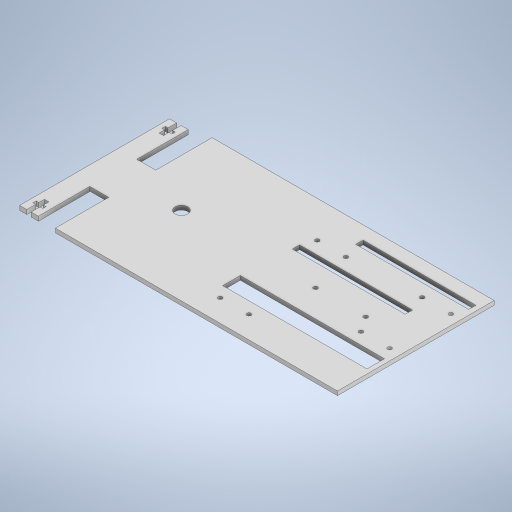
# Autodesk Inventor part: suelo_imp
Saved by Autodesk Inventor 2024 (Build 280153020, 153B)
## iProperties
Created: 2023-05-01
Part Number: suelo_imp
Material: Generic
Document SubType Name: Modeling
Designer: Diego
Density: 1 g/cm^3
Appearance: Default
Author: Diego
Autodesk Inventor part; units mm, degrees
ref_plane "YZ Plane" through (0, 0, 0) normal (1, 0, 0) x (0, 1, 0)
ref_plane "XZ Plane" through (0, 0, 0) normal (0, 1, 0) x (-1, 0, 0)
ref_plane "XY Plane" through (0, 0, 0) normal (0, 0, 1) x (1, 0, 0)
sketch "Sketch1" plane through (0, 0, 0) normal (0, 1, 0) x (-1, 0, 0)
  line L0 (-97.5, -62.5) -> (97.5, -62.5)
  line L1 (97.5, 62.5) -> (-97.5, 62.5)
  line L2 (-97.5, 62.5) -> (-97.5, -62.5)
  line L3 (-97.5, -62.5) -> (97.5, 62.5) construction
  line L4 (97.5, -62.5) -> (-97.5, 62.5) construction
  line L5 (97.5, 20) -> (112.525, 20)
  line L6 (127.475, 21.2237) -> (127.475, -18.7763)
  line L7 (112.525, -17.5526) -> (97.5, -17.5526)
  line L8 (97.5, -62.5) -> (97.5, -17.5526)
  line L9 (97.5, 20) -> (97.5, 62.5)
  line L10 (112.525, 20) -> (112.525, 61)
  line L11 (127.475, 61) -> (127.475, 21.2237)
  line L12 (127.475, 1.2237) -> (97.475, 1.2237) construction
  line L13 (112.525, -17.5526) -> (112.525, -58.5526)
  line L14 (127.475, -58.5526) -> (127.475, -18.7763)
  line L15 (119.975, 61) -> (121.775, 61) construction
  line L16 (118.225, 61) -> (118.225, 59)
  line L17 (119.975, 61) -> (119.975, 52.3078) construction
  line L18 (118.225, 59) -> (114.175, 59)
  line L19 (114.175, 59) -> (114.175, 56)
  line L20 (114.175, 56) -> (118.175, 56)
  line L21 (118.175, 56) -> (118.175, 53)
  line L22 (112.525, 61) -> (118.225, 61)
  line L23 (127.475, 61) -> (121.775, 61)
  line L24 (119.975, -58.5526) -> (121.775, -58.5526) construction
  line L25 (112.525, -58.5526) -> (118.225, -58.5526)
  line L26 (127.475, -58.5526) -> (121.775, -58.5526)
  line L27 (118.175, 53) -> (118.175, 47)
  line L28 (118.175, 47) -> (121.775, 47)
  line L29 (119.975, -58.5526) -> (121.775, -58.5526) construction
  line L30 (121.775, -58.5526) -> (121.775, -56.5526)
  line L31 (118.225, -58.5526) -> (118.225, -56.5526)
  line L32 (121.775, -56.5526) -> (125.775, -56.5526)
  line L33 (125.775, -56.5526) -> (125.775, -53.5526)
  line L34 (125.775, -53.5526) -> (121.775, -53.5526)
  line L35 (121.775, -58.5526) -> (121.775, -50.5526) construction
  line L36 (119.975, -58.5526) -> (119.975, -49.8604) construction
  line L37 (114.175, -53.5526) -> (118.175, -53.5526)
  line L38 (114.175, -56.5526) -> (114.175, -53.5526)
  line L39 (118.225, -56.5526) -> (114.175, -56.5526)
  line L40 (118.175, -53.5526) -> (118.175, -50.5526)
  line L41 (112.525, -58.5526) -> (118.225, -58.5526)
  line L42 (127.475, -58.5526) -> (121.775, -58.5526)
  line L43 (121.775, -53.5526) -> (121.775, -44.5526)
  line L44 (118.175, -50.5526) -> (118.175, -44.5526)
  line L45 (118.175, -44.5526) -> (121.775, -44.5526)
  line L46 (127.475, 61) -> (127.475, 79) construction
  line L47 (-97.5, 0) -> (-67.5, 0) construction
  line L48 (-67.5, 62.5) -> (-67.5, -62.5) construction
  line L49 (127.475, 79) -> (-67.5, 0) construction
  line L50 (127.475, -58.5526) -> (127.475, -76.5526) construction
  line L51 (127.475, -76.5526) -> (-67.5, 0) construction
  line L52 (-97.5, 62.5) -> (-117.5, 62.5)
  line L53 (-117.5, 62.5) -> (-117.5, -62.5)
  line L54 (-117.5, -62.5) -> (-97.5, -62.5)
  line L55 (-97.5, -62.5) -> (-97.5, 62.5)
  line L56 (-67.5, 0) -> (-47.5, 0) construction
  circle A0 centre (-47.5, 0) radius 1.6
  line L57 (-67.5, 0) -> (-87.5, 0) construction
  circle A1 centre (-87.5, 0) radius 1.6
  line L58 (121.775, 59.5898) -> (118.225, 59.5898) construction
  line L59 (121.775, 61) -> (121.775, 47)
  line L60 (121.775, 61) -> (121.775, 55) construction
  point P0 (0, 0)
  point P1 (121.775, 53)
  point P2 (121.775, -50.5526)
  point P3 (-97.5, -62.5)
  dimension "d0" = 195
  dimension "d1" = 125
  dimension "d3" = 30
  dimension "d4" = 40
  dimension "d5" = 15
  dimension "d6" = 41
  dimension "d11" = 7.5
  dimension "d12" = 1.8
  dimension "d13" = 1.75
  dimension "d15" = 2
  dimension "d21" = 30
  dimension "d22" = 8.6922
  dimension "d23" = 1.5
  dimension "d28" = 18
  dimension "d29" = 30
  dimension "d30" = 18
  dimension "d35" = 20
  dimension "d36" = 125
  dimension "d41" = 20
  dimension "d42" = 3.2
  dimension "d43" = 20
  dimension "d47" = 3.2
  dimension "d90" = 6
  constraints: 122 end point, 16 symmetric about line, 12 perpendicular, 7 horizontal, 7 point on line, 5 parallel, 5 vertical, 4 midpoint, 2 centre point, 2 coincident
  measures "d0" distance of L1.end L1.start
  measures "d1" distance of L1.start L0.end
  measures "d3" distance of L5.start L6.start
  measures "d4" distance of L6.start L6.end
  measures "d5" distance of L5.end L6.start
  measures "d6" distance of L5.end L10.end
  measures "d11" distance of L11.start L15.start
  measures "d12" distance of L15.end L15.start
  measures "d13" distance of L15.start L16.start
  measures "d15" distance of L16.start L16.end
  measures "d21" distance from line of L12.end L11
  measures "d22" distance from line of L17.end L23
  measures "d23" distance between parallel lines of L23 L1
  measures "d28" distance of L11.start L46.end
  measures "d29" distance of L47.start L47.end
  measures "d30" distance of L14.start L50.end
  measures "d35" distance of L54.end L53.end
  measures "d36" distance of L53.end L52.end
  measures "d41" distance of L47.end L56.end
  measures "d42" diameter of A0
  measures "d43" distance of L47.end L57.end
  measures "d47" diameter of A1
  measures "d90" distance of L15.end L60.end
extrude "Extrusion1" add sketch "Sketch1" along normal blind 3.25 contours L2 L1 L9 L5 L10 L22 L16 L18 L19 L20 L21 L27 L28 L59 L23 L11 L6 L14 L26 L30 L32 L33 L34 L43 L45 L44 L40 L37 L38 L39 L31 L25 L13 L7 L8 L0 | A0 | A1
sketch "Sketch2" plane through (0, 3.25, 0) normal (0, 1, 0) x (1, 0, 0)
  line L0 (-127.475, 58.5526) -> (-127.475, -61) construction
  line L1 (-127.475, 0) -> (-59.475, 0) construction
  circle A0 centre (-59.475, 0) radius 5
  point P0 (0, 0)
  dimension "d31" = 68
  dimension "d32" = 10
  constraints: 2 end point, 1 centre point, 1 coincident, 1 perpendicular, 1 point on line
  measures "d31" distance of L1.start L1.end
  measures "d32" diameter of A0
extrude "Extrusion2" cut sketch "Sketch2" against normal blind 10
sketch "Sketch3" plane through (97.5, 0, 62.5) normal (1, 0, 0) x (0, 0, -1)
  line L0 (125, 0) -> (80.0526, 0) projected
  line L1 (0, 3.25) -> (125, 3.25)
  line L2 (125, 3.25) -> (125, 0)
  line L3 (125, 0) -> (0, 0)
  line L4 (0, 0) -> (0, 3.25)
  point P0 (62.5, 0)
  constraints: 8 end point, 2 parallel, 1 horizontal, 1 perpendicular
extrude "Extrusion4" add sketch "Sketch3" along normal blind 30
extrude "Extrusion5" cut sketch "Sketch1" along normal blind 4 contours A0 | A1
sketch "Sketch4" plane through (0, 3.25, 0) normal (0, 1, 0) x (1, 0, 0)
  line L0 (-97.5, -62.5) -> (127.5, -62.5) construction
  line L1 (39.3, -62.5) -> (39.3, -44.9) construction
  line L2 (127.5, 62.5) -> (127.5, -62.5) construction
  circle A0 centre (39.3, -44.9) radius 1.6
  circle A1 centre (16.42, -44.9) radius 1.6
  line L3 (39.3, -44.9) -> (16.42, -44.9) construction
  line L4 (118.8, -62.5) -> (118.8, -12.2) construction
  circle A2 centre (118.8, -12.2) radius 1.6
  line L5 (118.8, -12.2) -> (95.92, -12.2) construction
  circle A3 centre (95.92, -12.2) radius 1.6
  line L6 (-97.5, 62.5) -> (127.5, 62.5) construction
  line L7 (119.5, 62.5) -> (119.5, 35.9) construction
  circle A4 centre (119.5, 35.9) radius 1.6
  line L8 (119.5, 35.9) -> (96.62, 35.9) construction
  circle A5 centre (96.62, 35.9) radius 1.6
  line L9 (38.32, 62.5) -> (38.32, 33.4) construction
  circle A6 centre (38.32, 33.4) radius 1.6
  line L10 (38.32, 33.4) -> (15.44, 33.4) construction
  circle A7 centre (15.44, 33.4) radius 1.6
  point P0 (0, 0)
  point P1 (119.5, 49.2)
  dimension "d48" = 88.2
  dimension "d49" = 17.6
  dimension "d50" = 3.2
  dimension "d51" = 3.2
  dimension "d52" = 22.88
  dimension "d53" = 50.3
  dimension "d54" = 8.7
  dimension "d55" = 3.2
  dimension "d56" = 3.2
  dimension "d57" = 22.88
  dimension "d58" = 8
  dimension "d59" = 26.6
  dimension "d60" = 3.2
  dimension "d61" = 22.88
  dimension "d62" = 3.2
  dimension "d63" = 89.18
  dimension "d64" = 29.1
  dimension "d65" = 3.2
  dimension "d66" = 22.88
  dimension "d67" = 3.2
  constraints: 16 end point, 8 centre point, 7 coincident, 4 point on line, 3 horizontal, 3 vertical, 2 perpendicular, 1 midpoint
  measures "d48" distance between parallel lines of L1 L2
  measures "d49" distance of L1.start L1.end
  measures "d50" diameter of A0
  measures "d51" diameter of A1
  measures "d52" distance of L3.start L3.end
  measures "d53" distance of L4.start L4.end
  measures "d54" distance between parallel lines of L2 L4
  measures "d55" diameter of A2
  measures "d56" diameter of A3
  measures "d57" distance of L5.start L5.end
  measures "d58" distance from line of L2 point (119.5, 49.2)
  measures "d59" distance of L7.start L7.end
  measures "d60" diameter of A4
  measures "d61" distance of L8.start L8.end
  measures "d62" diameter of A5
  measures "d63" distance between parallel lines of L2 L9
  measures "d64" distance of L9.start L9.end
  measures "d65" diameter of A6
  measures "d66" distance of L10.start L10.end
  measures "d67" diameter of A7
extrude "Extrusion6" cut sketch "Sketch4" against normal blind 10
sketch "Sketch5" plane through (0, 3.25, 0) normal (0, 1, 0) x (1, 0, 0)
  circle A0 centre (119.5, 35.9) radius 1.6 construction
  line L0 (123.5, 48.9829) -> (78.5, 48.9829) construction
  line L1 (123.5, 46.1029) -> (33.5, 46.1029)
  line L2 (33.5, 46.1029) -> (33.5, 51.8629)
  line L3 (33.5, 51.8629) -> (123.5, 51.8629)
  line L4 (123.5, 51.8629) -> (123.5, 46.1029)
  line L5 (123.5, 46.1029) -> (33.5, 51.8629) construction
  line L6 (33.5, 46.1029) -> (123.5, 51.8629) construction
  line L7 (127.5, 62.5) -> (127.5, -62.5) projected
  circle A1 centre (15.44, 33.4) radius 1.6 construction
  line L8 (11.5, 20.4) -> (56.5, 20.4) construction
  line L9 (101.5, 17.525) -> (11.5, 17.525)
  line L10 (11.5, 17.525) -> (11.5, 23.275)
  line L11 (11.5, 23.275) -> (101.5, 23.275)
  line L12 (101.5, 23.275) -> (101.5, 17.525)
  line L13 (101.5, 17.525) -> (11.5, 23.275) construction
  line L14 (11.5, 17.525) -> (101.5, 23.275) construction
  circle A2 centre (95.92, -12.2) radius 1.6 construction
  line L15 (111.5, -28.5) -> (66.5, -28.5) construction
  line L16 (124, -35.5) -> (9, -35.5)
  line L17 (9, -35.5) -> (9, -21.5)
  line L18 (9, -21.5) -> (124, -21.5)
  line L19 (124, -21.5) -> (124, -35.5)
  line L20 (124, -35.5) -> (9, -21.5) construction
  line L21 (9, -35.5) -> (124, -21.5) construction
  line L22 (-97.5, -62.5) -> (127.5, -62.5) projected
  point P0 (0, 0)
  dimension "d71" = 45
  dimension "d72" = 90
  dimension "d73" = 5.76
  dimension "d76" = 4
  dimension "d78" = 45
  dimension "d79" = 90
  dimension "d80" = 5.75
  dimension "d82" = 26
  dimension "d84" = 45
  dimension "d85" = 115
  dimension "d86" = 14
  dimension "d87" = 3.5
  dimension "d88" = 27
  constraints: 42 end point, 6 horizontal, 6 midpoint, 6 parallel, 3 perpendicular
  measures "d71" distance of L0.start L0.end
  measures "d72" distance of L2.end L3.end
  measures "d73" distance of L1.end L2.end
  measures "d76" distance between parallel lines of L7 L4
  measures "d78" distance of L8.start L8.end
  measures "d79" distance of L10.end L11.end
  measures "d80" distance of L9.end L10.end
  measures "d82" distance between parallel lines of L7 L12
  measures "d84" distance of L15.start L15.end
  measures "d85" distance of L17.end L18.end
  measures "d86" distance of L16.end L17.end
  measures "d87" distance between parallel lines of L7 L19
  measures "d88" distance between parallel lines of L16 L22
extrude "Extrusion7" cut sketch "Sketch5" against normal blind 10
sketch "Sketch6" plane through (0, 3.25, 0) normal (0, 1, 0) x (1, 0, 0)
  line L0 (-127.475, -61) -> (-121.775, -61) projected
  line L1 (-112.525, 17.5526) -> (-112.525, 58.5526) projected
  line L2 (-127.475, -61) -> (-112.525, -61)
  line L3 (-112.525, -61) -> (-112.525, 58.5526)
  line L4 (-112.525, 58.5526) -> (-127.475, 58.5526)
  line L5 (-127.475, 58.5526) -> (-127.475, -61)
  point P0 (0, 0)
  constraints: 8 end point, 2 parallel, 1 horizontal, 1 perpendicular
extrude "Extrusion8" add sketch "Sketch6" against normal blind 3.5
sketch "Sketch7" plane through (0, 3.25, 0) normal (0, 1, 0) x (1, 0, 0)
  line L0 (-112.525, -61) -> (-127.475, -61) construction
  line L1 (-120, -61) -> (-121.75, -61) construction
  line L2 (-120, -61) -> (-118.25, -61) construction
  line L3 (-121.75, -47) -> (-118.25, -47)
  line L4 (-120, -61) -> (-120, -55.8389) construction
  line L5 (-121.75, -54) -> (-123.95, -54)
  line L6 (-123.95, -54) -> (-123.95, -51.4)
  line L7 (-123.95, -51.4) -> (-121.75, -51.4)
  line L8 (-121.75, -61) -> (-121.75, -54)
  line L9 (-121.75, -51.4) -> (-121.75, -47)
  line L10 (-118.25, -47) -> (-121.75, -47)
  line L11 (-118.25, -54) -> (-116.05, -54)
  line L12 (-116.05, -54) -> (-116.05, -51.4)
  line L13 (-116.05, -51.4) -> (-118.25, -51.4)
  line L14 (-118.25, -61) -> (-118.25, -54)
  line L15 (-118.25, -51.4) -> (-118.25, -47)
  line L16 (-127.475, 58.5526) -> (-127.475, -61) construction
  line L17 (-127.475, -1.2237) -> (-119.125, -1.2237) construction
  line L18 (-121.75, 44.5526) -> (-118.25, 44.5526)
  line L19 (-120, 58.5526) -> (-120, 53.3915) construction
  line L20 (-121.75, 51.5526) -> (-123.95, 51.5526)
  line L21 (-123.95, 51.5526) -> (-123.95, 48.9526)
  line L22 (-123.95, 48.9526) -> (-121.75, 48.9526)
  line L23 (-121.75, 58.5526) -> (-121.75, 51.5526)
  line L24 (-121.75, 48.9526) -> (-121.75, 44.5526)
  line L25 (-118.25, 44.5526) -> (-121.75, 44.5526)
  line L26 (-118.25, 51.5526) -> (-116.05, 51.5526)
  line L27 (-116.05, 51.5526) -> (-116.05, 48.9526)
  line L28 (-116.05, 48.9526) -> (-118.25, 48.9526)
  line L29 (-118.25, 58.5526) -> (-118.25, 51.5526)
  line L30 (-118.25, 48.9526) -> (-118.25, 44.5526)
  line L31 (-121.75, -61) -> (-118.25, -61)
  line L32 (-121.75, 58.5526) -> (-118.25, 58.5526)
  line L33 (-112.525, 58.5526) -> (-112.525, -61) projected
  point P0 (0, 0)
  dimension "d93" = 1.75
  dimension "d94" = 1.75
  dimension "d95" = 14
  dimension "d96" = 3.5
  dimension "d97" = 2.2
  dimension "d98" = 7
  dimension "d99" = 2.6
  constraints: 62 end point, 22 symmetric about line, 4 vertical, 3 horizontal, 3 perpendicular, 2 midpoint, 2 point on line, 1 collinear
  measures "d93" distance of L1.start L1.end
  measures "d94" distance of L1.start L2.end
  measures "d95" distance of L1.end L3.start
  measures "d96" distance of L3.start L3.end
  measures "d97" distance of L5.start L5.end
  measures "d98" distance between parallel lines of L0 L5
  measures "d99" distance of L5.end L6.end
extrude "Extrusion9" cut sketch "Sketch7" against normal blind 3.5
body "Solid1"
